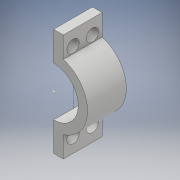
# Autodesk Inventor part: scopeCupler
Saved by Autodesk Inventor 2018 (Build 220112000, 112)
## iProperties
Created: 2019-03-22
Part Number: scopeCupler
Material: Generic
Document SubType Name: Modeling
Designer: Aditya Kendre
Density: 1 g/cm^3
Appearance: Default
Author: Aditya Kendre
Autodesk Inventor part; units mm, degrees
ref_plane "YZ Plane" through (0, 0, 0) normal (1, 0, 0) x (0, 1, 0)
ref_plane "XZ Plane" through (0, 0, 0) normal (0, 1, 0) x (-1, 0, 0)
ref_plane "XY Plane" through (0, 0, 0) normal (0, 0, 1) x (1, 0, 0)
sketch "Sketch1" plane through (0, 0, 0) normal (0, 1, 0) x (-1, 0, 0)
  circle A0 centre (0, 0) radius 12.7
  circle A1 centre (0, 0) radius 17.5
  dimension "d0" = 25.4
  dimension "d1" = 35
  constraints: 2 centre point, 2 coincident
  measures "d0" diameter of A0
  measures "d1" diameter of A1
extrude "Extrusion1" add sketch "Sketch1" along normal blind 20
sketch "Sketch2" plane through (0, 20, 0) normal (0, 1, 0) x (1, 0, 0)
  circle A0 centre (0, 0) radius 17.5 projected
  line L0 (0, -17.5) -> (-17.5, -17.5)
  line L1 (-17.5, -17.5) -> (-17.5, 18.3836)
  line L2 (-17.5, 18.3836) -> (0, 18.3836)
  line L3 (0, 18.3836) -> (0, -17.5)
  constraints: 8 end point, 2 parallel, 1 horizontal, 1 perpendicular, 1 vertical alignment, 1 other
extrude "Extrusion2" cut sketch "Sketch2" against normal blind 20 contours L0 L1 A0 | A0 L3 | L1 L2 L3 A0 picked at (-8.2181, -1.8757)
sketch "Sketch3" plane through (0, 20, 12.7) normal (-1, 0, 0) x (0, 0, 1)
  line L0 (-25.4, 0) -> (-25.4, -20) projected
  line L1 (-25.4, -20) -> (-40.4, -20)
  line L2 (-40.4, -20) -> (-40.4, 0)
  line L3 (-40.4, 0) -> (-25.4, 0)
  line L4 (-25.4, 0) -> (-25.4, -20)
  line L5 (-25.4, 0) -> (0, 0) projected
  line L6 (0, 0) -> (15, 0)
  line L7 (15, 0) -> (15, -20)
  line L8 (15, -20) -> (0, -20)
  line L9 (0, -20) -> (0, 0)
  point P0 (-12.7, -20)
  dimension "d6" = 15
  dimension "d7" = 15
  constraints: 16 end point, 4 parallel, 2 horizontal, 2 perpendicular, 1 point on line
  measures "d6" distance of L2.end L3.end
  measures "d7" distance of L7.end L8.end
sketch "Sketch4" plane through (0, 20, 12.7) normal (-1, 0, 0) x (0, 0, 1)
  line L0 (-25.4, 0) -> (-25.4, -20) construction
  line L1 (-25.4, -10) -> (-40.4302, -10) construction
  line L2 (-40.4302, -10) -> (15.0302, -10) construction
  point P0 (-12.7, -20)
  constraints: 4 end point, 1 horizontal, 1 midpoint, 1 point on line
extrude "Extrusion3" add sketch "Sketch3" against normal blind 5
sketch "Sketch5" plane through (0, 0, 12.7) normal (-1, 0, 0) x (0, 0, 1)
  line L0 (-29.4705, 0) -> (-40.4, 0) construction
  line L1 (-40.4, 0) -> (-25.4, 10) construction
  line L2 (-25.4, 20) -> (-25.4, 0) construction
  line L3 (-40.4, 10) -> (-25.4, 0) construction
  line L4 (-25.4, 0) -> (-40.4, 10) construction
  line L5 (-25.4, 20) -> (0, 20) construction
  line L6 (-40.4, 10) -> (-25.4, 20) construction
  line L7 (-25.4, 20) -> (-40.4, 20) construction
  line L8 (-40.4, 20) -> (-25.4, 10) construction
  line L9 (0, 0) -> (-25.4, 0) construction
  line L10 (0, 0) -> (15, 10) construction
  line L11 (15, 20) -> (15, 0) construction
  line L12 (0, 0) -> (0, 20) construction
  line L13 (0, 10) -> (15, 0) construction
  line L14 (0, 10) -> (15, 20) construction
  line L15 (0, 20) -> (15, 10) construction
  circle A0 centre (-32.9, 15) radius 3.175 construction
  circle A1 centre (-32.9, 15) radius 3.175
  circle A2 centre (-32.9, 5) radius 3.175
  circle A3 centre (7.5, 5) radius 3.175
  circle A4 centre (7.5, 15) radius 3.175
  point P0 (-12.7, 0)
  dimension "d10" = 6.35
  dimension "d11" = 6.35
  dimension "d12" = 6.35
  dimension "d13" = 6.35
  dimension "d14" = 6.35
  constraints: 20 end point, 7 midpoint, 5 centre point, 3 parallel, 2 collinear, 1 coincident
  measures "d10" diameter of A0
  measures "d11" diameter of A1
  measures "d12" diameter of A2
  measures "d13" diameter of A3
  measures "d14" diameter of A4
extrude "Extrusion4" cut sketch "Sketch5" against normal blind 5
body "Solid1"
